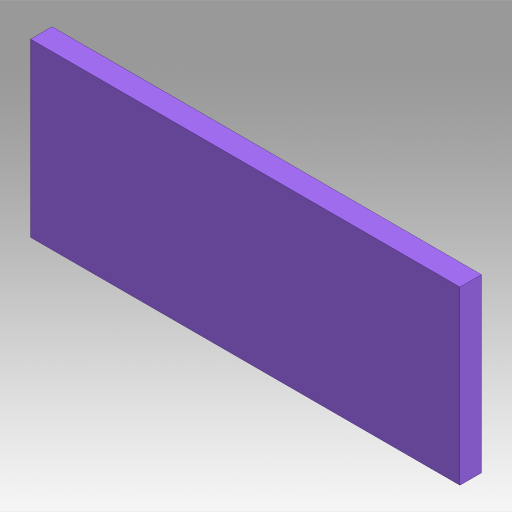
# Autodesk Inventor part: LEG_ATTACHMENT
Saved by Autodesk Inventor 2023 (Build 270158000, 158)
## iProperties
Created: 2025-04-08
Part Number: LEG_ATTACHMENT
Material: Steel, Mild
Document SubType Name: Modeling
Designer: NELLY NDUNG'U
Density: 7.85 g/cm^3
Appearance: Violet
Author: NELLY NDUNG'U
Autodesk Inventor part; units mm, degrees
ref_plane "YZ Plane" through (0, 0, 0) normal (1, 0, 0) x (0, 1, 0)
ref_plane "XZ Plane" through (0, 0, 0) normal (0, 1, 0) x (-1, 0, 0)
ref_plane "XY Plane" through (0, 0, 0) normal (0, 0, 1) x (1, 0, 0)
sketch "Sketch1" plane through (0, 0, 0) normal (1, 0, 0) x (0, 1, 0)
  line L0 (0, 0) -> (40, 0)
  line L1 (40, 0) -> (40, -5)
  line L2 (40, -5) -> (0, -5)
  line L3 (0, -5) -> (0, 0)
  dimension "d0" = 40
  dimension "d1" = 5
  constraints: 8 end point, 2 parallel, 1 horizontal, 1 perpendicular
  measures "d0" distance of L1.end L2.end
  measures "d1" distance of L0.end L1.end
extrude "Extrusion1" add sketch "Sketch1" along normal blind 100
body "Solid1"
